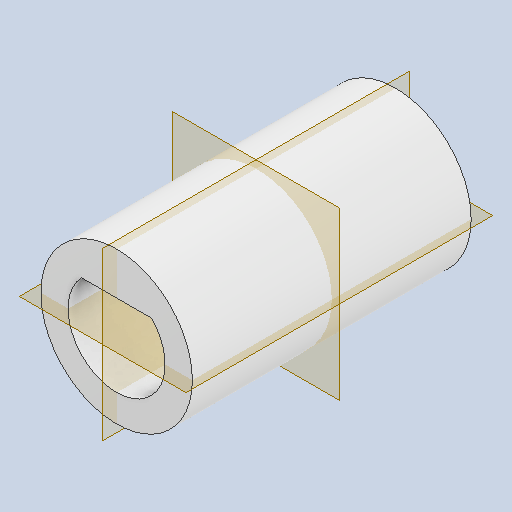
# Autodesk Inventor part: conector_motor_001
Saved by Autodesk Inventor 2026 (Build 300175000, 175)
## iProperties
Created: 2025-11-26
Part Number: conector_motor_001
Material: ABS Plastic
Document SubType Name: Modeling
Designer: Carlos Dias
Density: 1.06 g/cm^3
Appearance: Smooth - White
Author: Carlos Dias
Autodesk Inventor part; units mm, degrees
sketch "Sketch1" plane through (0, 0, 0) normal (0, 0, 1) x (1, 0, 0)
  circle A0 centre (0, 0) radius 2.5
  circle A1 centre (0, 0) radius 1.6 construction
  line L0 (-1.118, 1) -> (1.118, 1) projected
  arc A2 (-1.118, 1) -> (1.118, 1) centre (0, 0) ccw projected
  line L1 (-1.1619, 1.1) -> (1.1619, 1.1)
  arc A3 (-1.1619, 1.1) -> (1.1619, 1.1) centre (0, 0) ccw
  dimension "d1" = 3.2
  dimension "d0" = 5
  dimension "d4" = 0.5
  constraints: 2 centre point, 2 coincident, 2 end point, 2 point on circle, 1 horizontal, 5 other
  measures "d0" diameter of A0
extrude "Extrusion2" add sketch "Sketch1" along normal mid plane 9.2 contours A0
body "Solid2"
